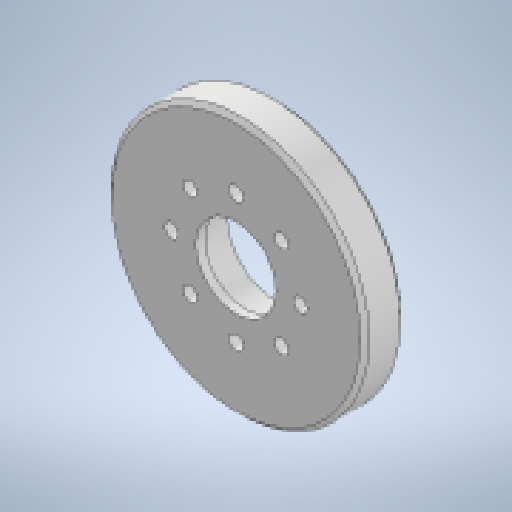
# Autodesk Inventor part: 内轮
Saved by Autodesk Inventor 2025.1 (Build 291241000, 241)
## iProperties
Created: 2025-08-27
Part Number: 内轮
Material: 常规
Document SubType Name: Modeling
Designer: Piw
Density: 1 g/cm^3
Appearance: 默认
Author: Piw
Autodesk Inventor part; units mm, degrees
ref_plane "YZ Plane" through (0, 0, 0) normal (1, 0, 0) x (0, 1, 0)
ref_plane "XZ Plane" through (0, 0, 0) normal (0, 1, 0) x (-1, 0, 0)
ref_plane "XY Plane" through (0, 0, 0) normal (0, 0, 1) x (1, 0, 0)
sketch "草图1" plane through (0, 0, 0) normal (0, 0, 1) x (1, 0, 0)
  circle A0 centre (0, 0) radius 28
  circle A1 centre (0, 0) radius 11
  dimension "d0" = 56
  dimension "d1" = 22
  constraints: 2 centre point, 2 coincident
  measures "d0" diameter of A0
  measures "d1" diameter of A1
extrude "拉伸1" add sketch "草图1" along normal blind 9
sketch "草图2" plane through (0, 0, 9) normal (0, 0, 1) x (1, 0, 0)
  circle A0 centre (0, 0) radius 28 projected
  circle A1 centre (0, 0) radius 9
  dimension "d4" = 18
  constraints: 1 centre point, 1 coincident
  measures "d4" diameter of A1
extrude "拉伸2" add sketch "草图2" along normal blind 2
sketch "草图3" plane through (0, 0, 11) normal (0, 0, 1) x (1, 0, 0)
  circle A0 centre (0, 0) radius 14.5 construction
  line L0 (-36.9419, 0) -> (43.6936, 0) construction
  circle A1 centre (14.5, 0) radius 1.6
  circle A2 centre (10.253, 10.253) radius 1.6
  circle A3 centre (0, 14.5) radius 1.6
  circle A4 centre (-10.253, 10.253) radius 1.6
  circle A5 centre (-14.5, 0) radius 1.6
  circle A6 centre (-10.253, -10.253) radius 1.6
  circle A7 centre (0, -14.5) radius 1.6
  circle A8 centre (10.253, -10.253) radius 1.6
  dimension "d7" = 29
  dimension "d8" = 3.2
  dimension "d11" = 360
  constraints: 8 centre point, 2 end point, 2 horizontal, 1 coincident, 1 horizontal alignment, 1 point on line, 19 other
  measures "d8" diameter of A1
extrude "拉伸3" cut sketch "草图3" against normal through all
chamfer "倒角1" distance 1 angle 45 2 edges at (-28, 0, 0) (-28, 0, 11)
sketch "草图4" plane through (0, 0, 0) normal (0, 0, -1) x (-1, 0, 0)
  circle A0 centre (0, 0) radius 19.5
  circle A1 centre (0, 0) radius 23
  dimension "d18" = 39
  dimension "d19" = 46
  constraints: 2 centre point, 2 coincident
  measures "d18" diameter of A0
  measures "d19" diameter of A1
extrude "拉伸4" cut sketch "草图4" against normal blind 2
chamfer "倒角2" distance 1 angle 45 2 edges at (23, 0, 0) (19.5, 0, 0)
sketch "草图5" plane through (0, 0, 0) normal (0, 0, -1) x (-1, 0, 0)
  circle A0 centre (0, 14.5) radius 1.6 projected
  circle A1 centre (0, 14.5) radius 3
  circle A2 centre (-10.253, 10.253) radius 3
  circle A3 centre (-14.5, 0) radius 3
  circle A4 centre (-10.253, -10.253) radius 3
  circle A5 centre (0, -14.5) radius 3
  circle A6 centre (10.253, -10.253) radius 3
  circle A7 centre (14.5, 0) radius 3
  circle A8 centre (10.253, 10.253) radius 3
  point P0 (0, 0)
  dimension "d25" = 6
  dimension "d28" = 360
  constraints: 8 centre point, 1 coincident, 17 other
  measures "d25" diameter of A1
extrude "拉伸5" cut sketch "草图5" against normal blind 3.5
